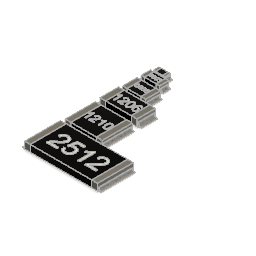
SMD Resistors (Autodesk Fusion 360 design; units mm, degrees)
Autodesk Fusion 360 part; units mm, degrees
sketch "Sketch1" plane through (0, 0, 0) normal (0, 1, 0) x (1, 0, 0)
  line L0 (0, 0) -> (1, 0)
  line L1 (1, 0) -> (1, -0.5)
  line L2 (1, -0.5) -> (0, -0.5)
  line L3 (0, -0.5) -> (0, 0)
  line L4 (0.2, 0) -> (0.8, 0)
  line L5 (0.8, 0) -> (0.8, -0.5)
  line L6 (0.8, -0.5) -> (0.2, -0.5)
  line L7 (0.2, -0.5) -> (0.2, 0)
  line L8 (0, -0.5) -> (0, 0)
  line L9 (0, 0) -> (-0.15, 0)
  line L10 (-0.15, 0) -> (-0.15, -0.5)
  line L11 (-0.15, -0.5) -> (0, -0.5)
  line L12 (0, -0.5) -> (0, 0)
  line L13 (0, -0.75) -> (1.6, -0.75)
  line L14 (1.6, -0.75) -> (1.6, -1.55)
  line L15 (1.6, -1.55) -> (0, -1.55)
  line L16 (0, -1.55) -> (0, -0.75)
  line L17 (0, -0.75) -> (0.3, -0.75)
  line L18 (0.3, -0.75) -> (0.3, -1.55)
  line L19 (0.3, -1.55) -> (0, -1.55)
  line L20 (0, -1.55) -> (0, -0.75)
  line L21 (1.6, -0.75) -> (1.3, -0.75)
  line L22 (1.3, -0.75) -> (1.3, -1.55)
  line L23 (1.3, -1.55) -> (1.6, -1.55)
  line L24 (1.6, -1.55) -> (1.6, -0.75)
  dimension "d1" = 1
  dimension "d2" = 0.5
  dimension "d7" = 0.5
  dimension "d8" = 0.15
  dimension "d19" = 1.6
  dimension "d20" = 0.8
  dimension "d21" = 0.3
  dimension "d22" = 0.8
  dimension "d23" = 0.3
  constraint horizontal L0
  constraint vertical L1
  constraint horizontal L2
  constraint vertical L3
  constraint coincident L0.start L3.end
  constraint horizontal L4
  constraint vertical L5
  constraint horizontal L6
  constraint vertical L7
  constraint coincident L2 L5.end
  constraint coincident L0 L4.start
  constraint vertical L8
  constraint horizontal L9
  constraint vertical L10
  constraint horizontal L11
  constraint vertical L12
  constraint horizontal L13
  constraint vertical L14
  constraint horizontal L15
  constraint vertical L16
  constraint horizontal L17
  constraint vertical L18
  constraint horizontal L19
  constraint vertical L20
  constraint horizontal L21
  constraint vertical L22
  constraint horizontal L23
  constraint vertical L24
  measures "d1" distance of L0.start L0.end
  measures "d2" distance of L0.start L2.end
  measures "d7" distance of L0.start L2.end
  measures "d8" distance of L0.start L9.end
  measures "d19" distance of L13.start L13.end
  measures "d20" distance of L13.start L15.end
  measures "d21" distance of L13.start L17.end
  measures "d22" distance of L13.end L14.end
  measures "d23" distance of L13.end L21.end
extrude "Extrude6" add sketch "Sketch1" along normal blind 0.5 contours L13 L15 L18 L22 makes body 1
extrude "Extrude1" add sketch "Sketch1" along normal blind 0.35 separate body contours L0 L2 L3 L7 L8 L12 | L0 L1 L2 L5 makes body 2 at (0, 0.1167, 0.3333) makes body 3 at (1, 0.1167, 0.1667)
extrude "Extrude2" add sketch "Sketch1" along normal blind 0.35 separate body contours L0 L2 L4 L5 L6 L7 makes body 4
sketch "Sketch2" plane through (0, 0, 0) normal (0, 1, 0) x (1, 0, 0)
  line L0 (-0.75, 0) -> (-0.5, 0)
  line L1 (-0.5, 0) -> (-0.5, -0.5)
  line L2 (-0.5, -0.5) -> (-0.75, -0.5)
  line L3 (-0.75, -0.5) -> (-0.75, 0)
  line L4 (-0.5089, 0) -> (-0.5, 0)
  line L5 (-0.5, 0) -> (-0.5, -0.5)
  line L6 (-0.5, -0.5) -> (-0.5089, -0.5)
  line L7 (-0.5089, -0.5) -> (-0.5089, 0)
  constraint horizontal L0
  constraint vertical L1
  constraint horizontal L2
  constraint vertical L3
  constraint horizontal L4
  constraint vertical L5
  constraint horizontal L6
  constraint vertical L7
  constraint coincident L0 L4.start
extrude "Extrude3" add sketch "Sketch2" along normal blind 0.25 separate body contours L0 L1 L2 L4 L5 L6 L7 makes body 5
extrude "Extrude4" add sketch "Sketch2" along normal blind 0.01 contours L0 L2 L3 L7 bodies 5
fillet "Fillet1" chord length 0.305 1 edges at (-0.5089, 0.01, 0.25) on bodies 5
fillet "Fillet2" chord length 0.095 6 edges at (-0.7373, 0.01, 0.5) (-0.572, 0.0732, 0.5) (-0.5089, 0.2378, 0.5) (-0.5089, 0.2378, 0) (-0.572, 0.0732, 0) (-0.7373, 0.01, 0) on bodies 5
fillet "Fillet3" radius 0.01 3 edges at (-0.75, 0.0075, 0.0489) (-0.75, 0.01, 0.25) (-0.75, 0.0075, 0.4511) on bodies 5
fillet "Fillet4" radius 0.008 3 edges at (-0.5066, 0.25, 0.0499) (-0.5089, 0.25, 0.25) (-0.5066, 0.25, 0.4501) on bodies 5
move_body "Move1" bodies 5 to x (1, 0, 0) y (0, 1, 0) z (0, 0, 1) at (0.5, 0.05, 0)
move_body "Move2" bodies 5 to x (1, 0, 0) y (0, 1, 0) z (0, 0, 1) at (0, -0.05, 0)
copy_body "CopyPasteBodies1" bodies 5 makes body 6
move_body "Move3" bodies 6 to x (-1, 0, 0) y (0, 1, 0) z (0, 0, -1) at (1, 0, 0.5)
sketch "Sketch3" plane through (0, 0.35, 0) normal (0, 1, 0) x (-1, 0, 0)
  line L0 (-0.2, 0.5) -> (-0.8, 0.5)
  line L1 (-0.8, 0.5) -> (-0.8, 0)
  line L2 (-0.8, 0) -> (-0.2, 0)
  line L3 (-0.2, 0) -> (-0.2, 0.5)
  line L4 (-0.2313, 0.3389) -> (-0.7639, 0.3389) construction
  line L5 (-0.7639, 0.3389) -> (-0.7639, 0.0889) construction
  line L6 (-0.7639, 0.0889) -> (-0.2313, 0.0889) construction
  line L7 (-0.2313, 0.0889) -> (-0.2313, 0.3389) construction
  text T0 "0402" font "Arial" height 0.25 align ink ink in box 0 x 0 at (-0.2313, 0.3389) x (-1, 0) y (0, -1) spacing 1 height is em
  constraint perpendicular L4 L5
  constraint parallel L4 L6
  constraint parallel L5 L7
extrude "Extrude5" add sketch "Sketch3" along normal blind 0.001 separate body text T0 makes body 7 at (0.4655, 0.35, 0.1873) makes body 8 at (0.535, 0.35, 0.2432) makes body 9 at (0.7052, 0.35, 0.3088) makes body 10 at (0.2569, 0.35, 0.2432)
extrude "Extrude7" add sketch "Sketch1" along normal blind 0.5 separate body contours L13 L15 L16 L17 L18 L19 L20 makes body 11
extrude "Extrude8" add sketch "Sketch1" along normal blind 0.5 separate body contours L13 L14 L15 L21 L22 L23 L24 makes body 12
sketch "Sketch4" plane through (0, 0, 0) normal (0, 1, 0) x (1, 0, 0)
  line L0 (-0.25, -1.55) -> (-0.26, -1.55)
  line L1 (-0.26, -1.55) -> (-0.26, -0.75)
  line L2 (-0.26, -0.75) -> (-0.25, -0.75)
  line L3 (-0.25, -0.75) -> (-0.25, -1.55)
  line L4 (-0.25, -0.75) -> (-0.5, -0.75)
  line L5 (-0.5, -0.75) -> (-0.5, -1.55)
  line L6 (-0.5, -1.55) -> (-0.25, -1.55)
  line L7 (-0.25, -1.55) -> (-0.25, -0.75)
  dimension "d30" = 0.8
  dimension "d31" = 0.01
  dimension "d32" = 0.25
  constraint horizontal L0
  constraint vertical L1
  constraint horizontal L2
  constraint vertical L3
  constraint horizontal L4
  constraint vertical L5
  constraint horizontal L6
  constraint vertical L7
  measures "d30" distance of L0.start L2.end
  measures "d31" distance of L0.start L0.end
  measures "d32" distance of L2.end L4.end
extrude "Extrude10" add sketch "Sketch4" along normal blind 0.3 contours L0 L1 L2 L3 L4 L6 L7 makes body 13
move_body "Move4" bodies 13 to x (1, 0, 0) y (0, 1, 0) z (0, 0, 1) at (0.25, 0.1, 0)
move_body "Move5" bodies 13 to x (1, 0, 0) y (0, 1, 0) z (0, 0, 1) at (0, -0.1, 0)
sketch "Sketch5" plane through (0, 0.5, 0) normal (0, 1, 0) x (-1, 0, 0)
  line L0 (-0.3, 0.75) -> (-0.3, 1.55)
  line L1 (-0.3, 1.55) -> (-1.3, 1.55)
  line L2 (-1.3, 1.55) -> (-1.3, 0.75)
  line L3 (-1.3, 0.75) -> (-0.3, 0.75)
  line L4 (-0.318, 1.3229) -> (-1.28, 1.3229) construction
  line L5 (-1.28, 1.3229) -> (-1.28, 0.8729) construction
  line L6 (-1.28, 0.8729) -> (-0.318, 0.8729) construction
  line L7 (-0.318, 0.8729) -> (-0.318, 1.3229) construction
  text T0 "0603" font "Arial" height 0.45 align ink ink in box 0 x 0 at (-0.318, 1.3229) x (-1, 0) y (0, -1) spacing 1 height is em
  constraint perpendicular L4 L5
  constraint parallel L4 L6
  constraint parallel L5 L7
extrude "Extrude11" add sketch "Sketch5" along normal blind 0.001 separate body text T0 makes body 14 at (0.5904, 0.5, 1.1254) makes body 15 at (0.8566, 0.5, 1.1666) makes body 16 at (1.2111, 0.5, 1.1234) makes body 17 at (0.356, 0.5, 1.1666)
sketch "Sketch6" plane through (0, 0, 0) normal (0, 1, 0) x (1, 0, 0)
  line L0 (-0.2, -1.9) -> (1.8, -1.9)
  line L1 (1.8, -1.9) -> (1.8, -3.15)
  line L2 (1.8, -3.15) -> (-0.2, -3.15)
  line L3 (-0.2, -3.15) -> (-0.2, -1.9)
  line L4 (-0.2, -1.9) -> (0.2, -1.9)
  line L5 (0.2, -1.9) -> (0.2, -3.15)
  line L6 (0.2, -3.15) -> (-0.2, -3.15)
  line L7 (-0.2, -3.15) -> (-0.2, -1.9)
  line L8 (1.8, -1.9) -> (1.4, -1.9)
  line L9 (1.4, -1.9) -> (1.4, -3.15)
  line L10 (1.4, -3.15) -> (1.8, -3.15)
  line L11 (1.8, -3.15) -> (1.8, -1.9)
  dimension "d43" = 2
  dimension "d44" = 1.25
  dimension "d45" = 0.4
  dimension "d46" = 1.25
  dimension "d47" = 0.4
  dimension "d48" = 1.25
  constraint horizontal L0
  constraint vertical L1
  constraint horizontal L2
  constraint vertical L3
  constraint horizontal L4
  constraint vertical L5
  constraint horizontal L6
  constraint vertical L7
  constraint horizontal L8
  constraint vertical L9
  constraint horizontal L10
  constraint vertical L11
  measures "d43" distance of L0.start L0.end
  measures "d44" distance of L0.start L2.end
  measures "d45" distance of L0.start L4.end
  measures "d46" distance of L0.start L2.end
  measures "d47" distance of L0.end L8.end
  measures "d48" distance of L0.end L1.end
extrude "Extrude12" add sketch "Sketch6" along normal blind 0.5 separate body contours L0 L2 L5 L9 makes body 18
extrude "Extrude13" add sketch "Sketch6" along normal blind 0.5 separate body contours L0 L1 L2 L8 L9 L10 L11 makes body 19
extrude "Extrude14" add sketch "Sketch6" along normal blind 0.5 separate body contours L0 L2 L3 L4 L5 L6 L7 makes body 20
sketch "Sketch7" plane through (0, 0, 0) normal (0, 1, 0) x (1, 0, 0)
  line L0 (-0.5, -1.9) -> (-0.51, -1.9)
  line L1 (-0.51, -1.9) -> (-0.51, -3.15)
  line L2 (-0.51, -3.15) -> (-0.5, -3.15)
  line L3 (-0.5, -3.15) -> (-0.5, -1.9)
  line L4 (-0.51, -1.9) -> (-0.76, -1.9)
  line L5 (-0.76, -1.9) -> (-0.76, -3.15)
  line L6 (-0.76, -3.15) -> (-0.51, -3.15)
  line L7 (-0.51, -3.15) -> (-0.51, -1.9)
  dimension "d55" = 1.25
  dimension "d56" = 0.01
  dimension "d57" = 0.25
  dimension "d58" = 1.25
  constraint horizontal L0
  constraint vertical L1
  constraint horizontal L2
  constraint vertical L3
  constraint horizontal L4
  constraint vertical L5
  constraint horizontal L6
  constraint vertical L7
  measures "d55" distance of L0.start L2.end
  measures "d56" distance of L0.start L0.end
  measures "d57" distance of L0.end L4.end
  measures "d58" distance of L0.end L1.end
sketch "Sketch8" plane through (-0.51, 0, 0) normal (-1, 0, 0) x (0, 0, 1)
  line L0 (3.0192, 0.3) -> (3.0192, 0.2928)
  line L1 (3.0192, 0.3) -> (2.0308, 0.3)
  line L2 (2.0308, 0.2928) -> (2.0308, 0.3)
  line L3 (3.0192, 0.2928) -> (2.0308, 0.2928)
sketch "Sketch9" plane through (0, 0.5, 0) normal (0, 1, 0) x (-1, 0, 0)
  line L0 (-0.2, 1.9) -> (-0.2, 3.15)
  line L1 (-0.2, 3.15) -> (-1.4, 3.15)
  line L2 (-1.4, 3.15) -> (-1.4, 1.9)
  line L3 (-1.4, 1.9) -> (-0.2, 1.9)
  line L4 (-0.2766, 2.6936) -> (-1.3482, 2.6936) construction
  line L5 (-1.3482, 2.6936) -> (-1.3482, 2.1936) construction
  line L6 (-1.3482, 2.1936) -> (-0.2766, 2.1936) construction
  line L7 (-0.2766, 2.1936) -> (-0.2766, 2.6936) construction
  text T0 "0805" font "Arial" height 0.5 align ink ink in box 0 x 0 at (-0.2766, 2.6936) x (-1, 0) y (0, -1) spacing 1 height is em
  constraint perpendicular L4 L5
  constraint parallel L4 L6
  constraint parallel L5 L7
extrude "Extrude18" add sketch "Sketch9" along normal blind 0.001 separate body text T0 makes body 21 at (0.7135, 0.5, 2.4739) makes body 22 at (0.8739, 0.5, 2.5223) makes body 23 at (1.2344, 0.5, 2.3284) makes body 24 at (0.3177, 0.5, 2.5223)
extrude "Extrude22" cut 1 faces at (-0.01, 0.1, 1.2833) along direction (1, 0, 0) blind 0.01 on bodies 13 bodies 13
extrude "Extrude23" add sketch "Sketch4" along normal blind 0.25 contours L0 L1 L2 L3 L4 L6 L7 bodies 13
extrude "Extrude24" add sketch "Sketch4" along normal blind 0.01 contours L1 L4 L5 L6 bodies 13
fillet "Fillet17" chord length 0.325 1 edges at (-0.26, 0.01, 1.15) on bodies 13
fillet "Fillet18" chord length 0.15 6 edges at (-0.4949, 0.01, 1.55) (-0.3273, 0.0773, 1.55) (-0.26, 0.2449, 1.55) (-0.26, 0.2449, 0.75) (-0.3273, 0.0773, 0.75) (-0.4949, 0.01, 0.75) on bodies 13
fillet "Fillet19" radius 0.01 3 edges at (-0.5, 0.0075, 0.833) (-0.5, 0.01, 1.15) (-0.5, 0.0075, 1.467) on bodies 13
fillet "Fillet20" radius 0.01 3 edges at (-0.2575, 0.25, 0.833) (-0.26, 0.25, 1.15) (-0.2575, 0.25, 1.467) on bodies 13
copy_body "CopyPasteBodies5" bodies 13 makes body 25
move_body "Move16" bodies 25 to x (1, 0, 0) y (0, 1, 0) z (0, 0, 1) at (2.3, 0, 0)
move_body "Move17" bodies 25 to x (-1, 0, 0) y (0, 1, 0) z (0, 0, -1) at (3.85, 0, 2.3)
move_body "Move18" bodies 13 to x (1, 0, 0) y (0, 1, 0) z (0, 0, 1) at (0.25, 0.125, 0)
move_body "Move19" bodies 13 to x (1, 0, 0) y (0, 1, 0) z (0, 0, 1) at (0, -0.125, 0)
move_body "Move20" bodies 25 to x (1, 0, 0) y (0, 1, 0) z (0, 0, 1) at (-0.2, 0.125, 0)
move_body "Move21" bodies 25 to x (1, 0, 0) y (0, 1, 0) z (0, 0, 1) at (0, -0.125, 0)
extrude "Extrude25" add sketch "Sketch7" along normal blind 0.25 separate body contours L0 L1 L2 L3 L7 makes body 26
extrude "Extrude26" add sketch "Sketch7" along normal blind 0.01 contours L1 L4 L5 L6 L7 bodies 26
fillet "Fillet21" chord length 0.335 1 edges at (-0.51, 0.01, 2.525) on bodies 26
fillet "Fillet22" chord length 0.155 6 edges at (-0.7534, 0.01, 3.15) (-0.5794, 0.0794, 3.15) (-0.51, 0.2484, 3.15) (-0.51, 0.2484, 1.9) (-0.5794, 0.0794, 1.9) (-0.7534, 0.01, 1.9) on bodies 26
fillet "Fillet23" radius 0.01 3 edges at (-0.5075, 0.25, 1.9862) (-0.51, 0.25, 2.525) (-0.5075, 0.25, 3.0638) on bodies 26
fillet "Fillet24" radius 0.01 3 edges at (-0.76, 0.0075, 1.9862) (-0.76, 0.01, 2.525) (-0.76, 0.0075, 3.0638) on bodies 26
move_body "Move23" bodies 26 to x (1, 0, 0) y (0, 1, 0) z (0, 0, 1) at (0.3, 0.125, 0)
copy_body "CopyPasteBodies7" bodies 26 makes body 27
move_body "Move24" bodies 27 to x (-0.999848, -0.017452, 0) y (-0.017452, 0.999848, 0) z (0, 0, -1) at (1.8599, -0.0091, 1.7998)
move_body "Move25" bodies 27 to x (1, 0, 0) y (0, 1, 0) z (0, 0, 1) at (-0.2555, 0.0056, 3.2502)
move_body "Move26" bodies 26 27 to x (1, 0, 0) y (0, 1, 0) z (0, 0, 1) at (0, -0.1, 0)
move_body "Move27" bodies 27 to x (1, 0, 0) y (0, 1, 0) z (0, 0, 1) at (0.0005, -0.0276, 0)
move_body "Move28" bodies 26 to x (1, 0, 0) y (0, 1, 0) z (0, 0, 1) at (0, -0.025, 0)
sketch "Sketch10" plane through (0, 0, 0) normal (0, 1, 0) x (1, 0, 0)
  line L0 (0, -3.5) -> (3.2, -3.5)
  line L1 (3.2, -3.5) -> (3.2, -5.1)
  line L2 (3.2, -5.1) -> (0, -5.1)
  line L3 (0, -5.1) -> (0, -3.5)
  line L4 (0, -3.5) -> (0.5, -3.5)
  line L5 (0.5, -3.5) -> (0.5, -5.1)
  line L6 (0.5, -5.1) -> (0, -5.1)
  line L7 (0, -5.1) -> (0, -3.5)
  line L8 (3.2, -3.5) -> (2.7, -3.5)
  line L9 (2.7, -3.5) -> (2.7, -5.1)
  line L10 (2.7, -5.1) -> (3.2, -5.1)
  line L11 (3.2, -5.1) -> (3.2, -3.5)
  dimension "d99" = 3.2
  dimension "d100" = 1.6
  dimension "d101" = 0.5
  dimension "d102" = 0.5
  constraint horizontal L0
  constraint vertical L1
  constraint horizontal L2
  constraint vertical L3
  constraint horizontal L4
  constraint vertical L5
  constraint horizontal L6
  constraint vertical L7
  constraint horizontal L8
  constraint vertical L9
  constraint horizontal L10
  constraint vertical L11
  measures "d99" distance of L0.start L0.end
  measures "d100" distance of L0.start L2.end
  measures "d101" distance of L0.start L4.end
  measures "d102" distance of L0.end L8.end
extrude "Extrude27" add sketch "Sketch10" along normal blind 0.6 separate body contours L0 L2 L5 L9 makes body 28
extrude "Extrude28" add sketch "Sketch10" along normal blind 0.6 separate body contours L0 L2 L3 L4 L5 L6 L7 makes body 29
extrude "Extrude29" add sketch "Sketch10" along normal blind 0.6 separate body contours L0 L1 L2 L8 L9 L10 L11 makes body 30
sketch "Sketch11" plane through (0, 0, 0) normal (0, 1, 0) x (1, 0, 0)
  line L0 (-0.5, -3.5) -> (-0.51, -3.5)
  line L1 (-0.51, -3.5) -> (-0.51, -5.1)
  line L2 (-0.51, -5.1) -> (-0.5, -5.1)
  line L3 (-0.5, -5.1) -> (-0.5, -3.5)
  line L4 (-0.5, -3.5) -> (-0.8, -3.5)
  line L5 (-0.8, -3.5) -> (-0.8, -5.1)
  line L6 (-0.8, -5.1) -> (-0.5, -5.1)
  line L7 (-0.5, -5.1) -> (-0.5, -3.5)
  dimension "d109" = 1.6
  dimension "d110" = 0.01
  dimension "d111" = 0.3
  dimension "d112" = 1.6
  constraint horizontal L0
  constraint vertical L1
  constraint horizontal L2
  constraint vertical L3
  constraint horizontal L4
  constraint vertical L5
  constraint horizontal L6
  constraint vertical L7
  measures "d109" distance of L0.start L2.end
  measures "d110" distance of L0.start L0.end
  measures "d111" distance of L0.start L4.end
  measures "d112" distance of L0.start L2.end
extrude "Extrude30" add sketch "Sketch11" along normal blind 0.3 separate body contours L0 L1 L2 L3 L4 L6 L7 makes body 31
extrude "Extrude31" add sketch "Sketch11" along normal blind 0.01 contours L1 L4 L5 L6 bodies 31
fillet "Fillet25" chord length 0.4 1 edges at (-0.51, 0.01, 4.3) on bodies 31
fillet "Fillet26" chord length 0.185 6 edges at (-0.7964, 0.01, 5.1) (-0.5929, 0.0928, 5.1) (-0.51, 0.2964, 5.1) (-0.51, 0.2964, 3.5) (-0.5928, 0.0929, 3.5) (-0.7964, 0.01, 3.5) on bodies 31
fillet "Fillet27" radius 0.01 3 edges at (-0.5075, 0.3, 3.6052) (-0.51, 0.3, 4.3) (-0.5075, 0.3, 4.9948) on bodies 31
fillet "Fillet28" radius 0.01 3 edges at (-0.8, 0.0075, 3.6052) (-0.8, 0.01, 4.3) (-0.8, 0.0075, 4.9948) on bodies 31
copy_body "CopyPasteBodies8" bodies 31 makes body 32
move_body "Move29" bodies 32 to x (1, 0, 0) y (0, 1, 0) z (0, 0, 1) at (4.5, 0, 0)
move_body "Move30" bodies 32 to x (-1, 0, 0) y (0, 1, 0) z (0, 0, -1) at (8, 0, 8.6)
move_body "Move31" bodies 31 to x (1, 0, 0) y (0, 1, 0) z (0, 0, 1) at (0.5, 0.15, 0)
move_body "Move32" bodies 32 to x (1, 0, 0) y (0, 1, 0) z (0, 0, 1) at (-0.8, 0.15, 0)
move_body "Move33" bodies 32 31 to x (1, 0, 0) y (0, 1, 0) z (0, 0, 1) at (0, -0.15, 0)
sketch "Sketch12" plane through (0, 0.6, 0) normal (0, 1, 0) x (-1, 0, 0)
  line L0 (-0.5, 3.5) -> (-0.5, 5.1)
  line L1 (-0.5, 5.1) -> (-2.7, 5.1)
  line L2 (-2.7, 5.1) -> (-2.7, 3.5)
  line L3 (-2.7, 3.5) -> (-0.5, 3.5)
  line L4 (-0.5528, 4.6869) -> (-2.6226, 4.6869) construction
  line L5 (-2.6226, 4.6869) -> (-2.6226, 3.6869) construction
  line L6 (-2.6226, 3.6869) -> (-0.5528, 3.6869) construction
  line L7 (-0.5528, 3.6869) -> (-0.5528, 4.6869) construction
  text T0 "1206" font "Arial" height 1 align ink ink in box 0 x 0 at (-0.5528, 4.6869) x (-1, 0) y (0, -1) spacing 1 height is em
  constraint perpendicular L4 L5
  constraint parallel L4 L6
  constraint parallel L5 L7
extrude "Extrude32" add sketch "Sketch12" along normal blind 0.001 separate body text T0 makes body 33 at (1.2387, 0.6, 4.6265) makes body 34 at (1.6699, 0.6, 4.3644) makes body 35 at (2.1907, 0.6, 4.2729) makes body 36 at (0.7972, 0.6, 4.2284)
sketch "Sketch13" plane through (0, 0, 0) normal (0, 1, 0) x (1, 0, 0)
  line L0 (0, -5.5) -> (3.2, -5.5)
  line L1 (3.2, -5.5) -> (3.2, -8.1)
  line L2 (3.2, -8.1) -> (0, -8.1)
  line L3 (0, -8.1) -> (0, -5.5)
  line L4 (0, -5.5) -> (0.5, -5.5)
  line L5 (0.5, -5.5) -> (0.5, -8.1)
  line L6 (0.5, -8.1) -> (0, -8.1)
  line L7 (0, -8.1) -> (0, -5.5)
  line L8 (3.2, -5.5) -> (2.7, -5.5)
  line L9 (2.7, -5.5) -> (2.7, -8.1)
  line L10 (2.7, -8.1) -> (3.2, -8.1)
  line L11 (3.2, -8.1) -> (3.2, -5.5)
  dimension "d123" = 2.6
  dimension "d124" = 0.5
  dimension "d125" = 0.5
  dimension "d126" = 2.6
  constraint horizontal L0
  constraint vertical L1
  constraint horizontal L2
  constraint vertical L3
  constraint horizontal L4
  constraint vertical L5
  constraint horizontal L6
  constraint vertical L7
  constraint vertical L9
  constraint horizontal L10
  constraint vertical L11
  measures "d123" distance of L0.start L2.end
  measures "d124" distance of L0.start L4.end
  measures "d125" distance of L0.end L8.end
  measures "d126" distance of L0.end L1.end
extrude "Extrude33" add sketch "Sketch13" along normal blind 0.5 separate body contours L0 L2 L5 L9 makes body 37
extrude "Extrude34" add sketch "Sketch13" along normal blind 0.5 separate body contours L0 L2 L3 L4 L5 L6 L7 makes body 38
extrude "Extrude35" add sketch "Sketch13" along normal blind 0.5 separate body contours L0 L1 L2 L8 L9 L10 L11 makes body 39
sketch "Sketch14" plane through (0, 0, 0) normal (0, 1, 0) x (1, 0, 0)
sketch "Sketch15" plane through (0, 0, 0) normal (0, 1, 0) x (1, 0, 0)
  line L0 (-0.5, -5.5) -> (-0.75, -5.5)
  line L1 (-0.75, -5.5) -> (-0.75, -8.1)
  line L2 (-0.75, -8.1) -> (-0.5, -8.1)
  line L3 (-0.5, -8.1) -> (-0.5, -5.5)
  line L4 (-0.5, -5.5) -> (-0.51, -5.5)
  line L5 (-0.51, -5.5) -> (-0.51, -8.1)
  line L6 (-0.51, -8.1) -> (-0.5, -8.1)
  line L7 (-0.5, -8.1) -> (-0.5, -5.5)
  dimension "d133" = 0.25
  dimension "d134" = 2.6
  dimension "d135" = 0.01
  dimension "d136" = 2.6
  constraint horizontal L0
  constraint vertical L1
  constraint horizontal L2
  constraint vertical L3
  constraint horizontal L4
  constraint vertical L5
  constraint horizontal L6
  constraint vertical L7
  measures "d133" distance of L0.start L0.end
  measures "d134" distance of L0.start L2.end
  measures "d135" distance of L0.start L4.end
  measures "d136" distance of L0.start L2.end
extrude "Extrude36" add sketch "Sketch15" along normal blind 0.25 separate body contours L0 L2 L3 L4 L5 L6 L7 makes body 40
extrude "Extrude37" add sketch "Sketch15" along normal blind 0.01 contours L0 L1 L2 L5 bodies 40
fillet "Fillet29" chord length 0.325 1 edges at (-0.51, 0.01, 6.8) on bodies 40
fillet "Fillet30" chord length 0.15 6 edges at (-0.7449, 0.01, 8.1) (-0.5773, 0.0773, 8.1) (-0.51, 0.2449, 8.1) (-0.51, 0.2449, 5.5) (-0.5773, 0.0773, 5.5) (-0.7449, 0.01, 5.5) on bodies 40
fillet "Fillet31" radius 0.01 3 edges at (-0.5075, 0.25, 5.583) (-0.51, 0.25, 6.8) (-0.5075, 0.25, 8.017) on bodies 40
fillet "Fillet32" radius 0.01 3 edges at (-0.75, 0.0075, 5.583) (-0.75, 0.01, 6.8) (-0.75, 0.0075, 8.017) on bodies 40
copy_body "CopyPasteBodies9" bodies 40 makes body 41
move_body "Move34" bodies 41 to x (1, 0, 0) y (0, 1, 0) z (0, 0, 1) at (4.9, 0, 0)
move_body "Move35" bodies 40 to x (1, 0, 0) y (0, 1, 0) z (0, 0, 1) at (0.5, 0.125, 0)
move_body "Move36" bodies 41 to x (-1, 0, 0) y (0, 1, 0) z (0, 0, -1) at (8.8, 0, 15.1708)
move_body "Move37" bodies 41 to x (1, 0, 0) y (0, 1, 0) z (0, 0, 1) at (-1.2, 0.125, -1.5708)
move_body "Move38" bodies 41 40 to x (1, 0, 0) y (0, 1, 0) z (0, 0, 1) at (0, -0.125, 0)
sketch "Sketch16" plane through (0, 0.5, 0) normal (0, 1, 0) x (-1, 0, 0)
  line L0 (-0.5, 5.5) -> (-0.5, 8.1)
  line L1 (-0.5, 8.1) -> (-2.7, 8.1)
  line L2 (-2.7, 8.1) -> (-2.7, 5.5)
  line L3 (-2.7, 5.5) -> (-0.5, 5.5)
  line L4 (-0.5571, 7.1637) -> (-2.625, 7.1637) construction
  line L5 (-2.625, 7.1637) -> (-2.625, 6.1637) construction
  line L6 (-2.625, 6.1637) -> (-0.5571, 6.1637) construction
  line L7 (-0.5571, 6.1637) -> (-0.5571, 7.1637) construction
  text T0 "1210" font "Arial" height 1 align ink ink in box 0 x 0 at (-0.5571, 7.1637) x (-1, 0) y (0, -1) spacing 1 height is em
  constraint perpendicular L4 L5
  constraint parallel L4 L6
  constraint parallel L5 L7
extrude "Extrude38" add sketch "Sketch16" along normal blind 0.001 separate body text T0 makes body 42 at (1.243, 0.5, 7.1034) makes body 43 at (1.9138, 0.5, 6.7053) makes body 44 at (2.2303, 0.5, 6.8412) makes body 45 at (0.8015, 0.5, 6.7053)
move_body "Move39" bodies 19 22 26 23 24 21 20 27 18 to x (1, 0, 0) y (0, 1, 0) z (0, 0, 1) at (0.2, 0, 0)
sketch "Sketch17" plane through (0, 0, 0) normal (0, 1, 0) x (1, 0, 0)
  line L0 (0, -8.5) -> (6.3, -8.5)
  line L1 (6.3, -8.5) -> (6.3, -11.6)
  line L2 (6.3, -11.6) -> (0, -11.6)
  line L3 (0, -11.6) -> (0, -8.5)
  line L4 (0, -8.5) -> (0.5, -8.5)
  line L5 (0.5, -8.5) -> (0.5, -11.6)
  line L6 (0.5, -11.6) -> (0, -11.6)
  line L7 (0, -11.6) -> (0, -8.5)
  line L8 (6.3, -8.5) -> (5.8, -8.5)
  line L9 (5.8, -8.5) -> (5.8, -11.6)
  line L10 (5.8, -11.6) -> (6.3, -11.6)
  line L11 (6.3, -11.6) -> (6.3, -8.5)
  dimension "d150" = 6.3
  dimension "d151" = 3.1
  dimension "d152" = 0.5
  dimension "d153" = 0.5
  dimension "d154" = 3.1
  constraint horizontal L0
  constraint vertical L1
  constraint horizontal L2
  constraint vertical L3
  constraint horizontal L4
  constraint vertical L5
  constraint horizontal L6
  constraint vertical L7
  constraint horizontal L8
  constraint vertical L9
  constraint horizontal L10
  constraint vertical L11
  measures "d150" distance of L0.start L0.end
  measures "d151" distance of L0.start L2.end
  measures "d152" distance of L0.start L4.end
  measures "d153" distance of L0.end L8.end
  measures "d154" distance of L0.end L1.end
extrude "Extrude39" add sketch "Sketch17" along normal blind 0.6 separate body contours L0 L2 L5 L9 makes body 46
extrude "Extrude40" add sketch "Sketch17" along normal blind 0.6 separate body contours L0 L2 L3 L4 L5 L6 L7 makes body 47
extrude "Extrude41" add sketch "Sketch17" along normal blind 0.6 separate body contours L0 L1 L2 L8 L9 L10 L11 makes body 48
sketch "Sketch18" plane through (0, 0, 0) normal (0, 1, 0) x (1, 0, 0)
  line L0 (-0.8, -8.5) -> (-0.55, -8.5)
  line L1 (-0.55, -8.5) -> (-0.55, -11.6)
  line L2 (-0.55, -11.6) -> (-0.8, -11.6)
  line L3 (-0.8, -11.6) -> (-0.8, -8.5)
  line L4 (-0.55, -8.5) -> (-0.56, -8.5)
  line L5 (-0.56, -8.5) -> (-0.56, -11.6)
  line L6 (-0.56, -11.6) -> (-0.55, -11.6)
  line L7 (-0.55, -11.6) -> (-0.55, -8.5)
  dimension "d162" = 0.25
  dimension "d163" = 3.1
  dimension "d164" = 0.01
  dimension "d165" = 3.1
  constraint horizontal L0
  constraint vertical L1
  constraint horizontal L2
  constraint vertical L3
  constraint horizontal L4
  constraint vertical L5
  constraint horizontal L6
  constraint vertical L7
  measures "d162" distance of L0.start L0.end
  measures "d163" distance of L0.start L2.end
  measures "d164" distance of L0.end L4.end
  measures "d165" distance of L0.end L1.end
extrude "Extrude42" add sketch "Sketch18" along normal blind 0.25 separate body contours L0 L1 L2 L4 L5 L6 L7 makes body 49
extrude "Extrude43" add sketch "Sketch18" along normal blind 0.01 contours L0 L2 L3 L5 bodies 49
fillet "Fillet33" chord length 0.335 1 edges at (-0.56, 0.01, 10.05) on bodies 49
fillet "Fillet34" chord length 0.155 6 edges at (-0.7984, 0.01, 11.6) (-0.6294, 0.0794, 11.6) (-0.56, 0.2484, 11.6) (-0.56, 0.2484, 8.5) (-0.6294, 0.0794, 8.5) (-0.7984, 0.01, 8.5) on bodies 49
fillet "Fillet35" radius 0.01 3 edges at (-0.5575, 0.25, 8.5862) (-0.56, 0.25, 10.05) (-0.5575, 0.25, 11.5138) on bodies 49
fillet "Fillet36" radius 0.01 3 edges at (-0.8, 0.0075, 8.5862) (-0.8, 0.01, 10.05) (-0.8, 0.0075, 11.5138) on bodies 49
copy_body "CopyPasteBodies10" bodies 49 makes body 50
move_body "Move40" bodies 50 to x (1, 0, 0) y (0, 1, 0) z (0, 0, 1) at (8, 0, 0)
move_body "Move41" bodies 50 to x (-1, 0, 0) y (0, 1, 0) z (0, 0, -1) at (14.9, 0, 21.2624)
move_body "Move42" bodies 50 to x (1, 0, 0) y (0, 1, 0) z (0, 0, 1) at (-1.15, 0.175, -1.1624)
move_body "Move43" bodies 49 to x (1, 0, 0) y (0, 1, 0) z (0, 0, 1) at (0.55, 0, 0)
move_body "Move44" bodies 50 to x (1, 0, 0) y (0, 1, 0) z (0, 0, 1) at (0, -0.175, 0)
sketch "Sketch19" plane through (0, 0.6, 0) normal (0, 1, 0) x (-1, 0, 0)
  line L0 (-0.5, 8.5) -> (-0.5, 11.6)
  line L1 (-0.5, 11.6) -> (-5.8, 11.6)
  line L2 (-5.8, 11.6) -> (-5.8, 8.5)
  line L3 (-5.8, 8.5) -> (-0.5, 8.5)
  line L4 (-1, 10.8029) -> (-5.2852, 10.8029) construction
  line L5 (-5.2852, 10.8029) -> (-5.2852, 8.8029) construction
  line L6 (-5.2852, 8.8029) -> (-1, 8.8029) construction
  line L7 (-1, 8.8029) -> (-1, 10.8029) construction
  text T0 "2512" font "Arial" height 2 align ink ink in box 0 x 0 at (-1, 10.8029) x (-1, 0) y (0, -1) spacing 1 height is em
  constraint perpendicular L4 L5
  constraint parallel L4 L6
  constraint parallel L5 L7
extrude "Extrude44" add sketch "Sketch19" along normal blind 0.001 separate body text T0 makes body 51 at (3.8607, 0.6, 9.906) makes body 52 at (4.7439, 0.6, 10.7022) makes body 53 at (2.599, 0.6, 9.4024) makes body 54 at (1.407, 0.6, 10.7022)
